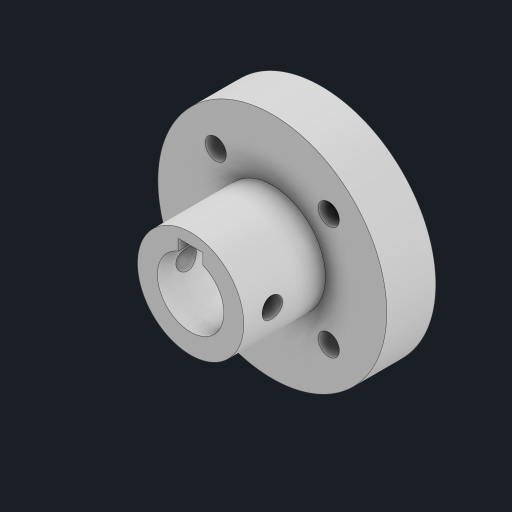
# Autodesk Inventor part: BaseHub
Saved by Autodesk Inventor 2023 (Build 270158000, 158)
## iProperties
Created: 2024-01-25
Part Number: BaseHub
Material: Generic
Document SubType Name: Modeling
Designer: valer
Density: 1 g/cm^3
Appearance: Default
Author: valer
Autodesk Inventor part; units mm, degrees
ref_plane "YZ Plane" through (0, 0, 0) normal (1, 0, 0) x (0, 1, 0)
ref_plane "XZ Plane" through (0, 0, 0) normal (0, 1, 0) x (-1, 0, 0)
ref_plane "XY Plane" through (0, 0, 0) normal (0, 0, 1) x (1, 0, 0)
sketch "Hub" plane through (0, 0, 0) normal (0, 0, 1) x (1, 0, 0)
  circle A0 centre (0, 0) radius 6.6 construction
  circle A1 centre (-6.9148, 6.9148) radius 1.5875 construction
  circle A2 centre (6.9148, 6.9148) radius 1.5875 construction
  circle A3 centre (-6.9148, -6.9148) radius 1.5875 construction
  circle A4 centre (6.9148, -6.9148) radius 1.5875 construction
  line L0 (-6.9148, 6.9148) -> (6.9148, 6.9148) construction
  line L1 (6.9148, 6.9148) -> (6.9148, -6.9148) construction
  line L2 (6.9148, -6.9148) -> (-6.9148, -6.9148) construction
  line L3 (-6.9148, -6.9148) -> (-6.9148, 6.9148) construction
  circle A5 centre (0, 0) radius 12.958 construction
  line L4 (-6.9148, -6.9148) -> (6.9148, 6.9148) construction
  line L5 (-6.9148, 6.9148) -> (-5.7923, 5.7923) construction
  line L6 (-5.7923, 5.7923) -> (-4.6669, 4.6669) construction
  line L7 (-8.0373, 8.0373) -> (-9.1627, 9.1627) construction
  circle A6 centre (0, 0) radius 4.0625
  line L8 (0, 4.0625) -> (0, 5.1125) construction
  line L9 (0, -21.9812) -> (0, 19.9969) construction
  line L10 (-1.5, 5.1125) -> (1.5, 5.1125)
  line L11 (-1.5, 5.1125) -> (-1.5, 3.7754)
  line L12 (1.5, 5.1125) -> (1.5, 3.7754)
  circle A7 centre (0, 0) radius 14
  circle A8 centre (6.9148, 6.9148) radius 1.2891
  circle A9 centre (6.9148, -6.9148) radius 1.2891
  circle A10 centre (-6.9148, -6.9148) radius 1.2891
  circle A11 centre (-6.9148, 6.9148) radius 1.2891
  circle A12 centre (6.9148, -6.9148) radius 2.84 construction
  circle A13 centre (12.3744, -12.3744) radius 1.621 construction
  circle A14 centre (12.3744, -12.3744) radius 3.61 construction
  dimension "d0" = 13.2
  dimension "d1" = 3.175
  dimension "d5" = 13.8296
  dimension "d6" = 45
  dimension "d9" = 8.125
  dimension "d10" = 1.05
  dimension "d11" = 3
  dimension "d21" = 2.5781
  dimension "d27" = 28
  dimension "d34" = 5.68
  dimension "d35" = 7.22
  constraints: 24 end point, 15 coincident, 12 centre point, 6 equal radius, 5 point on circle, 3 collinear, 3 vertical, 2 equal length, 2 horizontal, 2 midpoint, 2 parallel, 1 perpendicular, 6 other
  measures "d1" diameter of A1
  measures "d5" distance of L0.start L0.end
  measures "d6" angle of L0 L5
  measures "d9" diameter of A6
  measures "d10" distance of L8.end L8.start
  measures "d11" distance of L10.start L10.end
  measures "d21" diameter of A8
  measures "d27" diameter of A7
  measures "d34" diameter of A12
  measures "d35" diameter of A14
extrude "HubFeature" add sketch "Hub" against normal blind 6
sketch "Lip" plane through (0, 0, 0) normal (0, 0, 1) x (1, 0, 0)
  circle A0 centre (0, 0) radius 6.5
  arc A1 (-1.5, 3.7754) -> (1.5, 3.7754) centre (0, 0) ccw projected
  line L0 (1.5, 5.1125) -> (1.5, 3.7754) projected
  line L1 (-1.5, 5.1125) -> (1.5, 5.1125) projected
  line L2 (-1.5, 3.7754) -> (-1.5, 5.1125) projected
  dimension "d28" = 13
  constraints: 1 centre point, 1 coincident
  measures "d28" diameter of A0
extrude "LipFeature" add sketch "Lip" along normal blind 10
sketch "SetScrewHole" plane through (0, 0, 0) normal (1, 0, 0) x (0, 1, 0)
  line L0 (6.5, 10) -> (-6.5, 10) construction
  line L1 (0, 10) -> (0, 0) construction
  circle A0 centre (0, 6.5) radius 1.25
  dimension "d30" = 2.5
  dimension "d31" = 3.5
  constraints: 2 end point, 1 centre point, 1 midpoint, 1 point on line, 1 vertical
  measures "d30" diameter of A0
  measures "d31" distance from line of L0 A0.centre
extrude "SetScrewHoleFeature" cut sketch "SetScrewHole" along normal through all both and the other way through all
sketch "Sketch7" plane through (0, 0, -6) normal (0, 0, -1) x (-1, 0, 0)
  circle A0 centre (0, 0) radius 14 projected
  circle A1 centre (0, 0) radius 12
  dimension "d38" = 24
  constraints: 1 centre point
  measures "d38" diameter of A1
extrude "Extrusion6" cut sketch "Sketch7" against normal blind 3 contours A1
body "Solid1"
